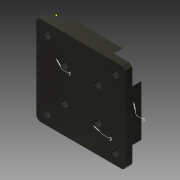
# Autodesk Inventor part: Bot
Saved by Autodesk Inventor 2015 (Build 190159000, 159)
## iProperties
Created: 2017-01-12
Part Number: Bot
Material: Generic
Document SubType Name: Modeling
Designer: Per
Density: 1 g/cm^3
Appearance: Gunmetal
Author: Per
Autodesk Inventor part; units mm, degrees
ref_plane "YZ Plane" through (0, 0, 0) normal (1, 0, 0) x (0, 1, 0)
ref_plane "XZ Plane" through (0, 0, 0) normal (0, 1, 0) x (-1, 0, 0)
ref_plane "XY Plane" through (0, 0, 0) normal (0, 0, 1) x (1, 0, 0)
sketch "Sketch1" plane through (0, 0, 0) normal (0, 1, 0) x (-1, 0, 0)
  line L0 (-36, -36) -> (0, -36)
  line L1 (0, -36) -> (0, 0)
  line L2 (-11.2353, -15.6026) -> (-15.4779, -11.36)
  line L3 (-15.4779, -7.1174) -> (-6.3606, 2)
  line L4 (2, -6.61) -> (-6.9926, -15.6026)
  circle A0 centre (-25.4718, -10.6529) radius 1.5
  line L5 (-15.4779, -7.1174) -> (-15.4779, -11.36)
  line L6 (-6.9926, -15.6026) -> (-11.2353, -15.6026)
  line L7 (-20.5221, -7.1174) -> (-29.6394, 2)
  line L8 (-38, -6.61) -> (-29.0074, -15.6026)
  line L9 (-24.7647, -15.6026) -> (-20.5221, -11.36)
  line L10 (-20.5221, -7.1174) -> (-20.5221, -11.36)
  line L11 (-29.0074, -15.6026) -> (-24.7647, -15.6026)
  line L12 (-15.4779, -28.8826) -> (-6.3606, -38)
  line L13 (2, -29.39) -> (-6.9926, -20.3974)
  line L14 (-11.2353, -20.3974) -> (-15.4779, -24.64)
  line L15 (-15.4779, -28.8826) -> (-15.4779, -24.64)
  line L16 (-6.9926, -20.3974) -> (-11.2353, -20.3974)
  line L17 (-20.5221, -28.8826) -> (-20.5221, -24.64)
  line L18 (-24.7647, -20.3974) -> (-20.5221, -24.64)
  line L19 (-20.5221, -28.8826) -> (-29.6394, -38)
  line L20 (-29.0074, -20.3974) -> (-24.7647, -20.3974)
  line L21 (-38, -29.39) -> (-29.0074, -20.3974)
  line L22 (0, 0) -> (-36, 0)
  line L23 (-36, 0) -> (-36, -36)
  circle A1 centre (-10.5282, -25.3471) radius 1.5
  circle A2 centre (-25.4718, -25.3471) radius 1.5
  circle A3 centre (-10.5282, -10.6529) radius 1.5
  line L24 (2, -38) -> (2, 2)
  line L25 (2, 2) -> (-38, 2)
  line L26 (-38, 2) -> (-38, -38)
  line L27 (-38, -38) -> (2, -38)
  circle A4 centre (-2.75, -2.75) radius 1.5
  circle A5 centre (-33.25, -2.75) radius 1.5
  circle A6 centre (-33.25, -33.25) radius 1.5
  circle A7 centre (-2.75, -33.25) radius 1.5
  point P0 (-9.114, -18.276)
  point P1 (-17.5992, -26.7613)
  point P2 (-26.886, -18.276)
  point P3 (-18.4008, -26.7613)
  point P4 (-9.114, -17.724)
  point P5 (-17.5992, -9.2387)
  point P6 (-18.4008, -9.2387)
  point P7 (-26.886, -17.724)
  dimension "d0" = 36
  dimension "d55" = 36
  dimension "d56" = 40
  dimension "d57" = 40
  dimension "d58" = 3
  dimension "d59" = 3
  dimension "d60" = 3
  dimension "d61" = 3
  constraints: 56 end point, 12 point on line, 8 centre point, 3 parallel, 2 perpendicular, 1 horizontal
  measures "d0" distance of L0.start L0.end
  measures "d55" distance of L0.start L23.start
  measures "d56" distance of L27.end L24.end
  measures "d57" distance of L26.start L24.end
  measures "d58" diameter of A4
  measures "d59" diameter of A5
  measures "d60" diameter of A6
  measures "d61" diameter of A7
extrude "Extrusion5" add sketch "Sketch1" along normal blind 3
extrude "Extrusion6" add sketch "Sketch1" along normal blind 7 contours L19 L17 L18 L20 L21 L23 L8 L11 L9 L10 L7 L22 L3 L5 L2 L6 L4 L1 L13 L16 L14 L15 L12 L0 | L0 L12 L27 L19 | L21 L26 L8 L23 | L1 L4 L24 L13 | L7 L25 L3 L22
fillet "Fillet2" radius 2 4 edges at (38, 1.5, 2) (-2, 1.5, 2) (-2, 1.5, -38) (38, 1.5, -38)
sketch "Sketch2" plane through (0, 7, 0) normal (0, 1, 0) x (1, 0, 0)
  circle A0 centre (1, 18) radius 1.5
  circle A1 centre (18, 35) radius 1.5
  circle A2 centre (35, 18) radius 1.5
  point P0 (0, 0)
  dimension "d56" = 40
  dimension "d68" = 3
  dimension "d71" = 3
  dimension "d72" = 3
  constraints: 3 centre point
  measures "d68" diameter of A0
  measures "d71" diameter of A1
  measures "d72" diameter of A2
body "Solid3"
